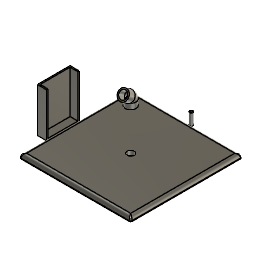
Top (Autodesk Fusion 360 design; units mm, degrees)
part number: 2026-02-08-13-54-52-596
Autodesk Fusion 360 part; units mm, degrees
sketch "Sketch1" plane through (0, 0, 0) normal (0, 0, 1) x (1, 0, 0)
  line L0 (-75, 50) -> (81, 50)
  line L1 (81, 50) -> (81, -106)
  line L2 (81, -106) -> (-75, -106)
  line L3 (-75, -106) -> (-75, 50)
  dimension "d1" = 156
  dimension "d2" = 156
  constraint horizontal L0
  constraint vertical L1
  constraint horizontal L2
  constraint vertical L3
  measures "d1" distance of L0.start L0.end
  measures "d2" distance of L0.start L2.end
extrude "Extrude1" add sketch "Sketch1" along normal blind 6 makes body 1
fillet "Fillet1" radius 2 4 edges at (81, -106, 3) (81, 50, 3) (-75, -106, 3) (-75, 50, 3) on bodies 1
fillet "Fillet2" radius 5 8 edges at (3, -106, 6) (-74.4142, -105.4142, 6) (-75, -28, 6) (-74.4142, 49.4142, 6) (3, 50, 6) (80.4142, 49.4142, 6) (81, -28, 6) (80.4142, -105.4142, 6) on bodies 1
sketch "Sketch2" plane through (0, 0, 6) normal (0, 0, 1) x (-1, 0, 0)
  line L0 (70, 101) -> (-76, 101)
  line L1 (-76, 101) -> (-76, -45)
  line L2 (-76, -45) -> (70, -45)
  line L3 (70, -45) -> (70, 101)
  circle A0 centre (-3, 28) radius 5
  dimension "d9" = 10
  dimension "d10" = 73
  dimension "d11" = 73
  measures "d9" diameter of A0
  measures "d10" distance of L3 A0.centre
  measures "d11" distance of L0 A0.centre
extrude "Extrude2" cut sketch "Sketch2" against normal blind 10 contours A0 bodies 1
sketch "Sketch3" plane through (0, 0, 6) normal (0, 0, 1) x (-1, 0, 0)
  circle A0 centre (-3, 28) radius 5
  line L0 (70, 101) -> (-76, 101)
  line L1 (-76, 101) -> (-76, -45)
  line L2 (-76, -45) -> (70, -45)
  line L3 (70, -45) -> (70, 101)
  circle A1 centre (-5, -55) radius 2.5
  dimension "d14" = 5
  measures "d14" diameter of A1
extrude "Extrude3" add sketch "Sketch3" along normal blind 16 separate body contours A1 makes body 2
move_body "Move1" bodies 2 to x (1, 0, 0) y (0, 1, 0) z (0, 0, 1) at (0, 0, -6)
sketch "Sketch4" plane through (0, 0, 16) normal (0, 0, 1) x (-1, 0, 0)
  circle A0 centre (-5, -55) radius 2.5
  circle A1 centre (-5, -55) radius 1.25
  dimension "d17" = 2.5
  constraint concentric A0 A1
  measures "d17" diameter of A1
extrude "Extrude4" cut sketch "Sketch4" against normal blind 8.8 contours A1 bodies 2
sketch "Sketch5" plane through (0, 0, 6) normal (0, 0, 1) x (-1, 0, 0)
  circle A0 centre (-3, 28) radius 5
  line L0 (70, 101) -> (-76, 101)
  line L1 (-76, 101) -> (-76, -45)
  line L2 (-76, -45) -> (70, -45)
  line L3 (70, -45) -> (70, 101)
  line L4 (110, 20) -> (97, 20)
  line L5 (97, 20) -> (97, 66)
  line L6 (97, 66) -> (110, 66)
  line L7 (110, 66) -> (110, 20)
  dimension "d20" = 13
  dimension "d21" = 46
  constraint horizontal L4
  constraint vertical L5
  constraint horizontal L6
  constraint vertical L7
  measures "d20" distance of L4.start L4.end
  measures "d21" distance of L4.start L6.end
extrude "Extrude5" add sketch "Sketch5" along normal blind 62 separate body contours L4 L5 L6 L7 makes body 3
sketch "Sketch6" plane through (0, 0, 68) normal (0, 0, 1) x (-1, 0, 0)
  line L0 (110, 66) -> (97, 66)
  line L1 (97, 66) -> (97, 20)
  line L2 (97, 20) -> (110, 20)
  line L3 (110, 20) -> (110, 66)
  line L4 (108, 22) -> (97, 22)
  line L5 (97, 22) -> (97, 64)
  line L6 (97, 64) -> (108, 64)
  line L7 (108, 64) -> (108, 22)
  dimension "d24" = 11
  dimension "d25" = 42
  constraint horizontal L4
  constraint vertical L5
  constraint horizontal L6
  constraint vertical L7
  measures "d24" distance of L4.start L4.end
  measures "d25" distance of L4.start L6.end
extrude "Extrude6" cut sketch "Sketch6" against normal blind 60 contours L1 L4 L5 L6 L7 bodies 3
move_body "Move2" bodies 3 to x (1, 0, 0) y (0, 1, 0) z (0, 0, 1) at (20, 0, -6)
sketch "Sketch8" plane through (0, 0, 0) normal (1, 0, 0) x (0, 1, 0)
  line L0 (30, 6) -> (30, 14)
  arc A0 (30, 14) -> (27.6841, 18.4489) centre (24.569, 14) ccw
  line L1 (27.6841, 18.4489) -> (19.4926, 24.1846)
  dimension "d30" = 55
  dimension "d31" = 10
  dimension "d42" = 8
  constraint vertical L0
  constraint tangent L0 A0
  constraint tangent A0 L1
  measures "d30" angle of L0 L1
  measures "d31" distance of A0.end L1.end
  measures "d42" distance of L0.start L0.end
move_body "Move3" bodies 1 2 3 to x (1, 0, 0) y (0, 1, 0) z (0, 0, 1) at (55, 0, 0)
sketch "Sketch9" plane through (0, 0, 6) normal (0, 0, 1) x (-1, 0, 0)
  circle A0 centre (-58, 28) radius 5
  line L0 (15, 101) -> (-131, 101)
  line L1 (-131, 101) -> (-131, -45)
  line L2 (-131, -45) -> (15, -45)
  line L3 (15, -45) -> (15, 101)
  circle A1 centre (0, -30) radius 5.5
  circle A2 centre (0, -30) radius 7.5
  dimension "d32" = 11
  dimension "d33" = 2
  measures "d32" diameter of A1
sweep "Sweep1" add profiles "Sketch9" path "Sketch8" along L0 A0 L1 section 1 contours A2 bodies 1
extrude "Extrude7" cut sketch "Sketch9" against normal blind 10 contours A1 bodies 1
move_body "Move4" bodies 1 2 3 to x (1, 0, 0) y (0, 1, 0) z (0, 0, 1) at (-55, 0, 0)
